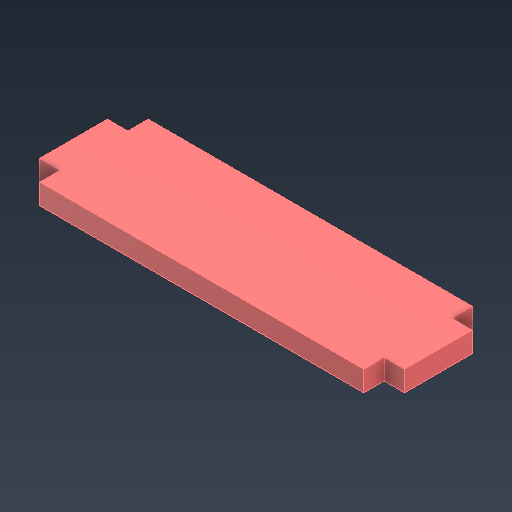
# Autodesk Inventor part: beam
Saved by Autodesk Inventor 2025.3 (Build 293356000, 356)
## iProperties
Created: 2025-09-04
Part Number: beam
Material: 木材 (楓木)
Document SubType Name: Modeling
Designer: 陳泓任
Density: 0.67 g/cm^3
Appearance: 平滑 - 紅色
Author: 陳泓任
Autodesk Inventor part; units mm, degrees
ref_plane "YZ Plane" through (0, 0, 0) normal (1, 0, 0) x (0, 1, 0)
ref_plane "XZ Plane" through (0, 0, 0) normal (0, 1, 0) x (-1, 0, 0)
ref_plane "XY Plane" through (0, 0, 0) normal (0, 0, 1) x (1, 0, 0)
sketch "草圖1" plane through (0, 0, 0) normal (0, 1, 0) x (-1, 0, 0)
  line L0 (0, 5) -> (3, 5)
  line L1 (3, 5) -> (3, 8)
  line L2 (50.7, 5) -> (53.7, 5)
  line L3 (50.7, -5) -> (53.7, -5)
  line L4 (50.7, -5) -> (50.7, -8)
  line L5 (3, -5) -> (3, -8)
  line L6 (0, -5) -> (3, -5)
  line L7 (3, -8) -> (50.7, -8)
  line L8 (53.7, -5) -> (53.7, 5)
  line L9 (50.7, 8) -> (3, 8)
  line L10 (0, 5) -> (0, -5)
  line L11 (0, 0) -> (0, -38.3248)
  line L12 (50.7, 5) -> (50.7, 8)
  dimension "d1" = 10
  dimension "d2" = 3
  dimension "d3" = 3
  dimension "d8" = 53.7
  constraints: 26 end point, 5 collinear, 4 equal length, 3 perpendicular, 2 parallel, 1 coincident, 1 midpoint, 1 vertical
  measures "d1" distance of L3.end L2.end
  measures "d2" distance of L0.end L1.end
  measures "d3" distance of L0.start L0.end
  measures "d8" distance between parallel lines of L10 L8
extrude "擠出1" add sketch "草圖1" along normal blind 3
